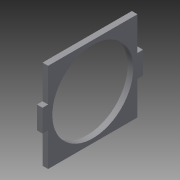
# Autodesk Inventor part: speakermount
Saved by Autodesk Inventor 2013 (Build 170138000, 138)
## iProperties
Created: 2013-07-18
Part Number: speakermount
Material: Generic
Document SubType Name: Modeling
Designer: owner
Density: 1 g/cm^3
Author: owner
Autodesk Inventor part; units mm, degrees
ref_plane "YZ Plane" through (0, 0, 0) normal (1, 0, 0) x (0, 1, 0)
ref_plane "XZ Plane" through (0, 0, 0) normal (0, 1, 0) x (-1, 0, 0)
ref_plane "XY Plane" through (0, 0, 0) normal (0, 0, 1) x (1, 0, 0)
sketch "Sketch1" plane through (0, 0, 0) normal (1, 0, 0) x (0, 1, 0)
  circle A0 centre (0, 0) radius 45.9994
  line L0 (-50.8, 0) -> (-50.8, 50.8)
  line L1 (-50.8, 0) -> (-50.8, -50.8)
  line L2 (-50.8, 50.8) -> (-12.7, 50.8)
  line L3 (-12.7, 50.8) -> (-12.7, 57.15)
  line L4 (-12.7, 57.15) -> (12.7, 57.15)
  line L5 (12.7, 57.15) -> (12.7, 50.8)
  line L6 (12.7, 50.8) -> (50.8, 50.8)
  line L7 (50.8, 50.8) -> (50.8, -50.8)
  line L8 (50.8, -50.8) -> (12.7, -50.8)
  line L9 (12.7, -50.8) -> (12.7, -57.15)
  line L10 (12.7, -57.15) -> (-12.7, -57.15)
  line L11 (-12.7, -57.15) -> (-12.7, -50.8)
  line L12 (-12.7, -50.8) -> (-50.8, -50.8)
  dimension "d0" = 91.9988
  dimension "d1" = 50.8
  dimension "d2" = 50.8
  dimension "d3" = 50.8
  dimension "d4" = 38.1
  dimension "d5" = 6.35
  dimension "d6" = 25.4
  dimension "d7" = 38.1
  dimension "d8" = 101.6
  dimension "d9" = 38.1
  dimension "d10" = 6.35
  dimension "d11" = 25.4
  dimension "d12" = 6.35
  constraints: 26 end point, 5 perpendicular, 4 parallel, 3 collinear, 1 centre point, 1 coincident
  measures "d0" diameter of A0
  measures "d1" distance of A0.centre L0.start
  measures "d2" distance of L0.start L0.end
  measures "d3" distance of L0.start L1.end
  measures "d4" distance of L0.end L2.end
  measures "d5" distance of L2.end L3.end
  measures "d6" distance of L3.end L4.end
  measures "d7" distance of L5.end L6.end
  measures "d8" distance of L6.end L7.end
  measures "d9" distance of L7.end L8.end
  measures "d10" distance of L8.end L9.end
  measures "d11" distance of L9.end L10.end
  measures "d12" distance of L10.end L11.end
extrude "Extrusion1" add sketch "Sketch1" along normal blind 6.35
body "Solid1"
